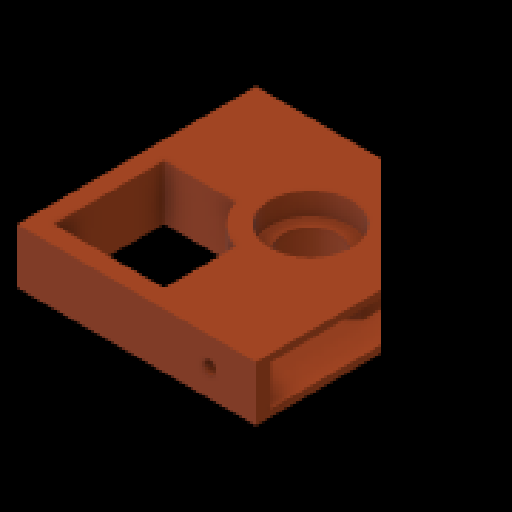
# Autodesk Inventor part: Z Axis Bottom Bearing Holder
Saved by Autodesk Inventor 2023.2 (Build 272271000, 271)
## iProperties
Created: 2023-02-17
Part Number: Z Axis Bottom Bearing Holder
Material: ABS Plastic
Document SubType Name: Modeling
Designer: remop
Density: 1.06 g/cm^3
Appearance: Smooth - Light Orange
Author: remop
Autodesk Inventor part; units mm, degrees
ref_plane "YZ Plane" through (0, 0, 0) normal (1, 0, 0) x (0, 1, 0)
ref_plane "XZ Plane" through (0, 0, 0) normal (0, 1, 0) x (-1, 0, 0)
ref_plane "XY Plane" through (0, 0, 0) normal (0, 0, 1) x (1, 0, 0)
sketch "Sketch1" plane through (0, 0, 0) normal (0, 1, 0) x (-1, 0, 0)
  line L0 (49.6871, 42.6052) -> (39.6871, 32.6052) projected
  line L1 (53.8292, 42.6052) -> (49.6871, 42.6052) projected
  line L2 (53.8292, 27.6052) -> (53.8292, 42.6052) projected
  line L3 (68.8292, 27.6052) -> (53.8292, 27.6052) projected
  line L4 (68.8292, 23.4631) -> (68.8292, 27.6052) projected
  line L5 (58.8292, 13.4631) -> (68.8292, 23.4631) projected
  line L6 (53.8292, 13.4631) -> (58.8292, 13.4631) projected
  line L7 (39.6871, 27.6052) -> (53.8292, 13.4631) projected
  line L8 (39.6871, 32.6052) -> (39.6871, 27.6052) projected
  line L9 (58.8292, 13.4631) -> (53.8292, 13.4631) projected
  line L10 (58.8292, 13.4631) -> (16.4028, -28.9633) projected
  line L11 (16.4028, -28.9633) -> (11.4028, -28.9633) projected
  line L12 (11.4028, -28.9633) -> (-2.7393, -14.8212) projected
  line L13 (-2.7393, -14.8212) -> (-2.7393, -9.8212) projected
  line L14 (-2.7393, -9.8212) -> (39.6871, 32.6052) projected
  line L15 (39.6871, 27.6052) -> (39.6871, 32.6052) projected
  line L16 (53.8292, 13.4631) -> (39.6871, 27.6052) projected
  circle A0 centre (13.9028, -12.3212) radius 11.15 projected
  line L17 (53.8292, 27.6052) -> (53.8292, -37.3948)
  line L18 (53.8292, 27.6052) -> (-11.1708, 27.6052)
  line L19 (53.8292, -37.3948) -> (49.8292, -37.3948)
  line L20 (49.8292, -37.3948) -> (49.8292, -12.3948)
  line L21 (49.8292, -12.3948) -> (32.9714, -12.3948)
  line L22 (-11.1708, 27.6052) -> (-11.1708, 23.6052)
  line L23 (-11.1708, 23.6052) -> (13.8292, 23.6052)
  line L24 (13.8292, 23.6052) -> (13.8292, 6.7473)
  point P0 (0, 0)
  dimension "d5" = 65
  dimension "d6" = 4
  dimension "d7" = 25
  constraints: 16 end point, 7 perpendicular, 2 horizontal, 2 point on line, 2 vertical
  measures "d5" distance of L2.start L18.end
  measures "d6" distance of L17.end L19.end
  measures "d7" distance of L22.end L23.end
extrude "Extrusion1" add sketch "Sketch1" against normal blind 15 contours L18 L17 L7 | L7 L17 L10 L11 L12 L13 L14 L18 | L14 L24 L23 L22 L18 | L17 L19 L20 L21 L10
sketch "Sketch2" plane through (0, -15, 0) normal (0, -1, 0) x (1, 0, 0)
  circle A0 centre (-13.9028, -12.3212) radius 11.15 projected
  circle A1 centre (-13.9028, -12.3212) radius 7.5
  point P0 (0, 0)
  dimension "d2" = 15
  constraints: 1 centre point, 1 coincident
  measures "d2" diameter of A1
extrude "Extrusion2" add sketch "Sketch2" against normal blind 9
sketch "Sketch3" plane through (0, 0, 0) normal (0, 1, 0) x (1, 0, 0)
  line L0 (2.7393, 14.8212) -> (-11.4028, 28.9633) projected
  line L1 (-11.4028, 28.9633) -> (-16.4028, 28.9633) projected
  line L2 (-16.4028, 28.9633) -> (-32.9714, 12.3948) projected
  line L3 (-32.9714, 12.3948) -> (-49.8292, 12.3948) projected
  line L4 (-49.8292, 12.3948) -> (-49.8292, 37.3948) projected
  line L5 (-49.8292, 37.3948) -> (-53.8292, 37.3948) projected
  line L6 (-53.8292, 37.3948) -> (-53.8292, -27.6052) projected
  line L7 (-53.8292, -27.6052) -> (11.1708, -27.6052) projected
  line L8 (11.1708, -27.6052) -> (11.1708, -23.6052) projected
  line L9 (11.1708, -23.6052) -> (-13.8292, -23.6052) projected
  line L10 (-13.8292, -23.6052) -> (-13.8292, -6.7473) projected
  line L11 (-13.8292, -6.7473) -> (2.7393, 9.8212) projected
  line L12 (2.7393, 9.8212) -> (2.7393, 14.8212) projected
  circle A0 centre (-13.9028, 12.3212) radius 11.15 projected
  line L13 (2.7393, 14.8212) -> (11.1708, 6.3898)
  line L14 (11.1708, 6.3898) -> (11.1708, -23.6052)
  line L15 (-11.4028, 28.9633) -> (-19.8343, 37.3948)
  line L16 (-19.8343, 37.3948) -> (-49.8292, 37.3948)
  line L17 (-11.4028, 28.9633) -> (-16.4028, 28.9633) projected
  point P0 (0, 0)
  constraints: 8 end point, 2 collinear, 1 parallel, 1 vertical
extrude "Extrusion3" add sketch "Sketch3" against normal blind 2 contours L13 L14 L9 L10 L11 L12 | L1 L2 L3 L4 L16 L15
sketch "Sketch4" plane through (0, -15, 0) normal (0, -1, 0) x (1, 0, 0)
  line L0 (2.7393, -9.8212) -> (-13.8292, 6.7473) projected
  line L1 (2.7393, -14.8212) -> (2.7393, -9.8212) projected
  line L2 (2.7393, -14.8212) -> (11.1708, -6.3898) projected
  line L3 (11.1708, -6.3898) -> (11.1708, 23.6052) projected
  line L4 (-13.8292, 23.6052) -> (11.1708, 23.6052) projected
  line L5 (-13.8292, 6.7473) -> (-13.8292, 23.6052) projected
  line L6 (-49.8292, -37.3948) -> (-19.8343, -37.3948) projected
  line L7 (-19.8343, -37.3948) -> (-11.4028, -28.9633) projected
  line L8 (-16.4028, -28.9633) -> (-11.4028, -28.9633) projected
  line L9 (-32.9714, -12.3948) -> (-16.4028, -28.9633) projected
  line L10 (-49.8292, -12.3948) -> (-32.9714, -12.3948) projected
  line L11 (-49.8292, -37.3948) -> (-49.8292, -12.3948) projected
  point P0 (0, 0)
extrude "Extrusion4" add sketch "Sketch4" against normal blind 2
sketch "Sketch5" plane through (11.1708, -2, 23.6052) normal (0, 0, -1) x (-1, 0, 0)
  line L0 (0, -11) -> (25, -11) projected
  line L1 (25, 0) -> (25, -11) projected
  line L2 (25, 0) -> (0, 0) projected
  line L3 (0, 0) -> (0, -11) projected
  point P0 (11.1708, 2)
  point P1 (12.5, -5.5)
  point P2 (0, -5.5)
  point P3 (12.5, 0)
  constraints: 2 midpoint, 1 horizontal alignment, 1 vertical alignment
hole "Hole1" at (-1.3292, -7.5, 23.6052) direction (0, 0, 1) diameter 3.5 end through all
sketch "Sketch6" plane through (-49.8292, -2, -12.3948) normal (1, 0, 0) x (0, 0, -1)
  line L0 (0, -11) -> (25, -11) projected
  line L1 (25, 0) -> (25, -11) projected
  line L2 (25, 0) -> (0, 0) projected
  line L3 (0, 0) -> (0, -11) projected
  point P0 (-12.3948, 2)
  point P1 (12.5, -5.5)
  point P2 (25, -5.5)
  point P3 (12.5, 0)
  constraints: 2 midpoint, 1 horizontal alignment, 1 vertical alignment
hole "Hole2" at (-49.8292, -7.5, -24.8948) direction (-1, 0, 0) diameter 3.5 end through all
sketch "Sketch7" plane through (0, 0, 0) normal (0, 1, 0) x (1, 0, 0)
  line L0 (11.1708, 6.3898) -> (-19.8343, 37.3948) projected
  line L1 (-19.8343, 37.3948) -> (-53.8292, 37.3948) projected
  line L2 (-53.8292, 37.3948) -> (-53.8292, -27.6052) projected
  line L3 (-53.8292, -27.6052) -> (11.1708, -27.6052) projected
  line L4 (11.1708, -27.6052) -> (11.1708, 6.3898) projected
  circle A0 centre (-13.9028, 12.3212) radius 11.15 projected
  line L5 (-48.8292, -22.6052) -> (-48.8292, 7.3948)
  circle A1 centre (-13.9028, 12.3212) radius 16.15
  line L6 (-48.8292, -22.6052) -> (-18.8292, -22.6052)
  line L7 (-18.8292, -22.6052) -> (-18.8292, -3.0591)
  line L8 (-48.8292, 7.3948) -> (-29.2831, 7.3948)
  point P0 (0, 0)
  dimension "d26" = 5
  dimension "d27" = 5
  dimension "d28" = 5
  dimension "d31" = 30
  constraints: 8 end point, 2 horizontal, 2 perpendicular, 2 point on circle, 1 centre point, 1 coincident, 1 vertical
  measures "d26" radial gap between concentric circles of A1 A0
  measures "d27" distance between parallel lines of L3 L6
  measures "d28" distance between parallel lines of L2 L5
  measures "d31" distance of L5.start L5.end
extrude "Extrusion5" cut sketch "Sketch7" against normal through all contours A1 L7 L6 L5 L8
equation "\"d27\" = d28"
body "Solid1"
